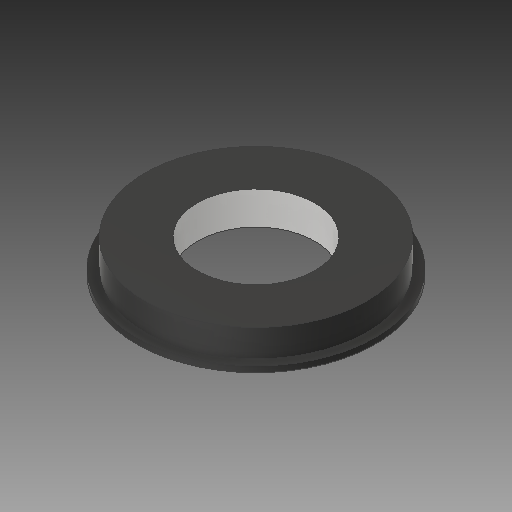
# Autodesk Inventor part: 큰 기어
Saved by Autodesk Inventor 2018 (Build 220112000, 112)
## iProperties
Created: 2018-04-03
Part Number: 큰 기어
Material: 일반
Document SubType Name: Modeling
Designer: CK
Density: 1 g/cm^3
Appearance: 기본값
Mass: 15.8974 g
Surface Area: 67.5087 cm^2
Volume: 15.8974 cm^3
Author: CK
Autodesk Inventor part; units mm, degrees
ref_plane "YZ Plane" through (0, 0, 0) normal (1, 0, 0) x (0, 1, 0)
ref_plane "XZ Plane" through (0, 0, 0) normal (0, 1, 0) x (-1, 0, 0)
ref_plane "XY Plane" through (0, 0, 0) normal (0, 0, 1) x (1, 0, 0)
sketch "스케치4" plane through (0, 0, 0) normal (0, 1, 0) x (-1, 0, 0)
  circle A0 centre (0, 0) radius 30.5
  circle A1 centre (0, 0) radius 15
  dimension "d8" = 61
  dimension "d9" = 30
  constraints: 2 centre point, 2 coincident
  measures "d8" diameter of A0
  measures "d9" diameter of A1
extrude "돌출3" add sketch "스케치4" along normal blind 8.45
sketch "스케치5" plane through (0, 8.45, 0) normal (0, 1, 0) x (1, 0, 0)
  circle A0 centre (0, 0) radius 28.3
  circle A1 centre (0, 0) radius 30.5
  dimension "d12" = 56.6
  constraints: 2 centre point, 2 coincident
  measures "d12" diameter of A0
extrude "돌출4" cut sketch "스케치5" against normal blind 6.95
